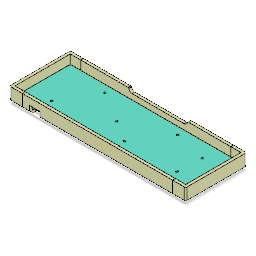
MiniVan_SpaceCut (Autodesk Fusion 360 design; units mm, degrees)
Autodesk Fusion 360 part; units mm, degrees
(part 1 of 4)
sketch "minivan_universal_plate_mount" plane through (80, 0, 0) normal (0, 1, 0) x (1, 0, 0)
  line L0 (-146.007, 0.6305) -> (-145.207, 0.6305)
  line L1 (-20.869, -43.7204) -> (-21.6683, -43.7204)
  line L2 (-243.231, -56.6448) -> (-243.231, 13.555101)
  line L3 (-146.007, 2.3007) -> (-146.007, 0.6305)
  line L4 (-137.022586, -19.0203) -> (-131.206, -19.0203)
  line L5 (-4.20028, -37.4695) -> (-4.20028, -24.6704)
  line L6 (-2.61827, -56.5195) -> (-1.81901, -56.5195)
  line L7 (-130.405, 0.6305) -> (-130.405, 2.3007)
  line L8 (-154.307, 7.53034) -> (-154.307, 4.7302)
  line L9 (-1.81901, -43.7204) -> (-2.61827, -43.7204)
  line L10 (-19.0004, -38.0703) -> (-4.99953, -38.0703)
  line L11 (-131.207, 0.6305) -> (-130.405, 0.6305)
  arc A0 (-243.231, 13.555101) -> (-240.231, 16.555101) centre (-240.231, 13.555101) cw
  line L12 (-153.432, 1.3) -> (-151.806, 1.3)
  line L13 (-130.405, -5.6203) -> (-131.206, -5.6203)
  line L14 (-17.4184, -56.5195) -> (-16.6192, -56.5195)
  line L15 (-151.806, 14.78019) -> (-151.806, 14.0004)
  line L16 (-1.81901, -56.5195) -> (-1.81901, -43.7204)
  line L17 (-145.205, -5.6203) -> (-146.006, -5.6203)
  line L18 (-151.806, 1.3) -> (-151.806, 0.1795)
  line L19 (-129.632, 1.3) -> (-127.905, 1.3)
  line L20 (-4.99953, -24.6704) -> (-4.99953, -24.0696)
  line L21 (-19.7997, -24.6704) -> (-19.7997, -37.4695)
  line L22 (-35.669, -43.7204) -> (-36.4684, -43.7204)
  line L23 (-24.5622, -18.4195) -> (-23.7629, -18.4195)
  line L24 (-9.76341, -19.0203) -> (-9.76341, -18.4195)
  line L25 (-19.0004, -37.4695) -> (-19.0004, -38.0703)
  line L26 (-36.4684, -43.7204) -> (-36.4684, -56.5195)
  line L27 (-36.4684, -56.5195) -> (-35.669, -56.5195)
  line L28 (-23.7629, -5.6203) -> (-24.5622, -5.6203)
  line L29 (-8.96278, -18.4195) -> (-8.96278, -5.6203)
  line L30 (-40.4301, -24.6704) -> (-41.2309, -24.6704)
  line L31 (-21.6683, -43.7204) -> (-21.6683, -43.1196)
  line L32 (-19.0004, -24.0696) -> (-19.0004, -24.6704)
  line L33 (-9.76341, -5.6203) -> (-9.76341, -5.0195)
  line L34 (-21.6683, -43.1196) -> (-30.570286, -43.1196)
  line L35 (-4.99953, -24.0696) -> (-19.0004, -24.0696)
  arc A1 (-30.570286, -42.918008) -> (-30.570286, -38.271592) centre (-31.493707, -40.5948) ccw
  line L36 (-25.6301, -24.6704) -> (-26.4308, -24.6704)
  line L37 (-26.4308, -24.0696) -> (-40.4301, -24.0696)
  line L38 (-21.6683, -56.5195) -> (-20.869, -56.5195)
  line L39 (-32.417127, -42.918008) -> (-32.417127, -43.1196)
  line L40 (-9.76341, -18.4195) -> (-8.96278, -18.4195)
  line L41 (-4.20028, -24.6704) -> (-4.99953, -24.6704)
  line L42 (-19.7997, -37.4695) -> (-19.0004, -37.4695)
  line L43 (-30.570286, -38.271592) -> (-30.570286, -38.0703)
  line L44 (-23.7629, -19.0203) -> (-9.76341, -19.0203)
  line L45 (-8.96278, -5.6203) -> (-9.76341, -5.6203)
  line L46 (-30.570286, -43.1196) -> (-30.570286, -42.918008)
  line L47 (-35.669, -56.5195) -> (-35.669, -57.1203)
  line L48 (-32.417127, -43.1196) -> (-35.669, -43.1196)
  line L49 (-24.5622, -5.6203) -> (-24.5622, -18.4195)
  line L50 (-30.570286, -38.0703) -> (-26.4308, -38.0703)
  line L51 (-26.4308, -37.4695) -> (-25.6301, -37.4695)
  line L52 (-4.99953, -38.0703) -> (-4.99953, -37.4695)
  line L53 (-9.76341, -5.0195) -> (-23.7629, -5.0195)
  line L54 (-26.4308, -38.0703) -> (-26.4308, -37.4695)
  line L55 (-21.6683, -57.1203) -> (-21.6683, -56.5195)
  line L56 (-25.6301, -37.4695) -> (-25.6301, -24.6704)
  line L57 (-35.669, -43.1196) -> (-35.669, -43.7204)
  line L58 (-35.669, -57.1203) -> (-21.6683, -57.1203)
  line L59 (-40.4301, -24.0696) -> (-40.4301, -24.6704)
  line L60 (-23.7629, -5.0195) -> (-23.7629, -5.6203)
  line L61 (-23.7629, -18.4195) -> (-23.7629, -19.0203)
  line L62 (-26.4308, -24.6704) -> (-26.4308, -24.0696)
  line L63 (-20.869, -56.5195) -> (-20.869, -43.7204)
  line L64 (-4.99953, -37.4695) -> (-4.20028, -37.4695)
  line L65 (-74.5684, -56.5195) -> (-73.769, -56.5195)
  line L66 (-82.7814, -37.4695) -> (-82.7814, -24.6704)
  arc A2 (-32.417127, -38.271592) -> (-32.417127, -42.918008) centre (-31.493707, -40.5948) ccw
  line L67 (-55.397707, 0.6305) -> (-54.598707, 0.6305)
  line L68 (-45.4822, -38.0703) -> (-45.4822, -37.4695)
  line L69 (-55.0058, -19.0203) -> (-55.0058, -18.4195)
  line L70 (-54.719, -56.5195) -> (-54.719, -57.1203)
  line L71 (-54.598707, 0.6305) -> (-54.598707, 0)
  line L72 (-35.1551, -18.4195) -> (-35.1551, -5.6203)
  line L73 (-49.9551, -19.0203) -> (-35.9558, -19.0203)
  line L74 (-54.719, -57.1203) -> (-40.7183, -57.1203)
  line L75 (-21.627707, 0.6305) -> (-20.828707, 0.6305)
  line L76 (-35.9558, -18.4195) -> (-35.1551, -18.4195)
  line L77 (-88.0551, -5.6203) -> (-88.8559, -5.6203)
  line L78 (-54.598707, 0) -> (-21.627707, 0)
  line L79 (-20.828707, 0.6305) -> (-20.828707, 13.42971)
  line L80 (-55.397707, 13.42971) -> (-55.397707, 0.6305)
  line L81 (-83.5808, -24.6704) -> (-83.5808, -24.0696)
  line L82 (-54.598707, 14.03054) -> (-54.598707, 13.42971)
  line L83 (-49.9551, -18.4195) -> (-49.9551, -19.0203)
  line L84 (-35.1551, -5.6203) -> (-35.9558, -5.6203)
  line L85 (-21.627707, 13.42971) -> (-21.627707, 14.03054)
  line L86 (-32.417127, -38.0703) -> (-32.417127, -38.271592)
  line L87 (-73.769, -56.5195) -> (-73.769, -57.1203)
  line L88 (-55.5184, -56.5195) -> (-54.719, -56.5195)
  line L89 (-55.0058, -18.4195) -> (-54.205, -18.4195)
  line L90 (-40.7183, -43.7204) -> (-40.7183, -43.1196)
  line L91 (-60.2823, -37.4695) -> (-59.4815, -37.4695)
  line L92 (-97.5801, -37.4695) -> (-97.5801, -38.0703)
  line L93 (-50.7559, -18.4195) -> (-49.9551, -18.4195)
  line L94 (-45.4822, -37.4695) -> (-44.6814, -37.4695)
  line L95 (-41.2309, -24.6704) -> (-41.2309, -37.4695)
  line L96 (-55.5184, -43.7204) -> (-55.5184, -56.5195)
  line L97 (-44.6814, -37.4695) -> (-44.6814, -24.6704)
  line L98 (-35.9558, -5.6203) -> (-35.9558, -5.0195)
  line L99 (-44.6814, -24.6704) -> (-45.4822, -24.6704)
  line L100 (-83.5808, -38.0703) -> (-83.5808, -37.4695)
  line L101 (-64.5322, -38.0703) -> (-64.5322, -37.4695)
  line L102 (-40.7183, -43.1196) -> (-54.719, -43.1196)
  line L103 (-73.255, -18.4195) -> (-73.255, -5.6203)
  line L104 (-49.9551, -5.0195) -> (-49.9551, -5.6203)
  line L105 (-40.4301, -37.4695) -> (-40.4301, -38.0703)
  line L106 (-49.9551, -5.6203) -> (-50.7559, -5.6203)
  line L107 (-39.9189, -43.7204) -> (-40.7183, -43.7204)
  line L108 (-21.627707, 0) -> (-21.627707, 0.6305)
  line L109 (-40.7183, -56.5195) -> (-39.9189, -56.5195)
  line L110 (-54.598707, 13.42971) -> (-55.397707, 13.42971)
  line L111 (-21.627707, 14.03054) -> (-54.598707, 14.03054)
  line L112 (-92.819, -57.1203) -> (-78.8183, -57.1203)
  line L113 (-50.7559, -5.6203) -> (-50.7559, -18.4195)
  line L114 (-41.2309, -37.4695) -> (-40.4301, -37.4695)
  line L115 (-35.9558, -19.0203) -> (-35.9558, -18.4195)
  line L116 (-54.719, -43.7204) -> (-55.5184, -43.7204)
  line L117 (-54.719, -43.1196) -> (-54.719, -43.7204)
  line L118 (-83.5808, -37.4695) -> (-82.7814, -37.4695)
  line L119 (-60.2823, -24.6704) -> (-60.2823, -37.4695)
  line L120 (-55.0058, -5.6203) -> (-55.0058, -5.0195)
  line L121 (-69.8059, -5.6203) -> (-69.8059, -18.4195)
  line L122 (-39.9189, -56.5195) -> (-39.9189, -43.7204)
  line L123 (-97.5801, -38.0703) -> (-83.5808, -38.0703)
  line L124 (-82.7814, -24.6704) -> (-83.5808, -24.6704)
  line L125 (-54.205, -5.6203) -> (-55.0058, -5.6203)
  line L126 (-54.205, -18.4195) -> (-54.205, -5.6203)
  line L127 (-98.3809, -37.4695) -> (-97.5801, -37.4695)
  line L128 (-97.5801, -24.0696) -> (-97.5801, -24.6704)
  line L129 (-59.7683, -57.1203) -> (-59.7683, -56.5195)
  line L130 (-69.0051, -5.0195) -> (-69.0051, -5.6203)
  line L131 (-73.255, -5.6203) -> (-74.0558, -5.6203)
  line L132 (-58.9689, -43.7204) -> (-59.7683, -43.7204)
  line L133 (-74.0558, -5.6203) -> (-74.0558, -5.0195)
  line L134 (-73.769, -43.1196) -> (-73.769, -43.7204)
  line L135 (-74.0558, -18.4195) -> (-73.255, -18.4195)
  line L136 (-78.5315, -24.6704) -> (-79.3309, -24.6704)
  line L137 (-92.819, -43.7204) -> (-93.6184, -43.7204)
  line L138 (-79.3309, -24.6704) -> (-79.3309, -37.4695)
  line L139 (-78.0189, -43.7204) -> (-78.8183, -43.7204)
  line L140 (-59.7683, -43.7204) -> (-59.7683, -43.1196)
  line L141 (-107.906, -5.6203) -> (-107.906, -18.4195)
  line L142 (-79.3309, -37.4695) -> (-78.5315, -37.4695)
  line L143 (-88.0551, -19.0203) -> (-74.0558, -19.0203)
  line L144 (-64.5322, -37.4695) -> (-63.7314, -37.4695)
  line L145 (-83.5808, -24.0696) -> (-97.5801, -24.0696)
  line L146 (-107.105, -5.6203) -> (-107.906, -5.6203)
  line L147 (-58.9689, -56.5195) -> (-58.9689, -43.7204)
  line L148 (-73.769, -57.1203) -> (-59.7683, -57.1203)
  line L149 (-93.6184, -43.7204) -> (-93.6184, -56.5195)
  line L150 (-64.5322, -24.0696) -> (-78.5315, -24.0696)
  line L151 (-74.0558, -5.0195) -> (-88.0551, -5.0195)
  line L152 (-78.8183, -43.7204) -> (-78.8183, -43.1196)
  line L153 (-63.7314, -37.4695) -> (-63.7314, -24.6704)
  line L154 (-74.5684, -43.7204) -> (-74.5684, -56.5195)
  line L155 (-78.5315, -37.4695) -> (-78.5315, -38.0703)
  line L156 (-64.5322, -24.6704) -> (-64.5322, -24.0696)
  line L157 (-88.0551, -5.0195) -> (-88.0551, -5.6203)
  line L158 (-88.0551, -18.4195) -> (-88.0551, -19.0203)
  line L159 (-88.8559, -18.4195) -> (-88.0551, -18.4195)
  line L160 (-108.825381, -38.0703) -> (-108.825381, -38.365605)
  line L161 (-116.918, -43.7204) -> (-116.918, -43.1196)
  line L162 (-78.8183, -57.1203) -> (-78.8183, -56.5195)
  line L163 (-116.918, -57.1203) -> (-116.918, -56.5195)
  line L164 (-101.83, -37.4695) -> (-101.83, -24.6704)
  line L165 (-126.155, -5.0195) -> (-126.155, -5.6203)
  line L166 (-116.119, -56.5195) -> (-116.119, -43.7204)
  line L167 (-131.718, -56.5195) -> (-130.919, -56.5195)
  line L168 (-97.8683, -43.1196) -> (-106.562032, -43.1196)
  line L169 (-126.956, -5.6203) -> (-126.956, -18.4195)
  line L170 (-93.1058, -18.4195) -> (-92.305, -18.4195)
  line L171 (-112.156, -19.0203) -> (-112.156, -18.4195)
  line L172 (-108.825381, -43.1196) -> (-111.869, -43.1196)
  line L173 (-92.819, -56.5195) -> (-92.819, -57.1203)
  line L174 (-117.431, -37.4695) -> (-116.63, -37.4695)
  line L175 (-74.0558, -19.0203) -> (-74.0558, -18.4195)
  line L176 (-130.919, -57.1203) -> (-116.918, -57.1203)
  line L177 (-92.819, -43.1196) -> (-92.819, -43.7204)
  line L178 (-107.906, -18.4195) -> (-107.105, -18.4195)
  line L179 (-98.3809, -24.6704) -> (-98.3809, -37.4695)
  line L180 (-111.869, -43.1196) -> (-111.869, -43.7204)
  line L181 (-111.869, -57.1203) -> (-97.8683, -57.1203)
  line L182 (-130.919, -43.7204) -> (-131.718, -43.7204)
  line L183 (-78.5315, -38.0703) -> (-64.5322, -38.0703)
  line L184 (-112.156, -5.0195) -> (-126.155, -5.0195)
  line L185 (-63.7314, -24.6704) -> (-64.5322, -24.6704)
  line L186 (-55.0058, -5.0195) -> (-69.0051, -5.0195)
  line L187 (-112.156, -18.4195) -> (-111.355, -18.4195)
  line L188 (-130.919, -56.5195) -> (-130.919, -57.1203)
  line L189 (-78.0189, -56.5195) -> (-78.0189, -43.7204)
  line L190 (-111.355, -18.4195) -> (-111.355, -5.6203)
  line L191 (-111.355, -5.6203) -> (-112.156, -5.6203)
  line L192 (-116.918, -56.5195) -> (-116.119, -56.5195)
  line L193 (-97.0689, -43.7204) -> (-97.8683, -43.7204)
  line L194 (-117.431, -24.6704) -> (-117.431, -37.4695)
  line L195 (-107.105, -19.0203) -> (-93.1058, -19.0203)
  line L196 (-97.5801, -24.6704) -> (-98.3809, -24.6704)
  line L197 (-106.562032, -43.1196) -> (-106.562032, -42.823995)
  line L198 (-78.8183, -56.5195) -> (-78.0189, -56.5195)
  line L199 (-73.769, -43.7204) -> (-74.5684, -43.7204)
  line L200 (-88.8559, -5.6203) -> (-88.8559, -18.4195)
  line L201 (-131.718, -43.7204) -> (-131.718, -56.5195)
  line L202 (-78.5315, -24.0696) -> (-78.5315, -24.6704)
  line L203 (-93.6184, -56.5195) -> (-92.819, -56.5195)
  line L204 (-93.1058, -5.0195) -> (-107.105, -5.0195)
  line L205 (-59.7683, -43.1196) -> (-73.769, -43.1196)
  line L206 (-116.63, -37.4695) -> (-116.63, -38.0703)
  line L207 (-112.668, -43.7204) -> (-112.668, -56.5195)
  arc A3 (-108.825381, -38.365605) -> (-108.825381, -42.823995) centre (-107.693707, -40.5948) ccw
  line L208 (-107.105, -18.4195) -> (-107.105, -19.0203)
  line L209 (-59.7683, -56.5195) -> (-58.9689, -56.5195)
  line L210 (-106.562032, -38.0703) -> (-102.631, -38.0703)
  line L211 (-102.631, -37.4695) -> (-101.83, -37.4695)
  line L212 (-116.63, -24.6704) -> (-117.431, -24.6704)
  line L213 (-106.562032, -38.365605) -> (-106.562032, -38.0703)
  line L214 (-108.825381, -42.823995) -> (-108.825381, -43.1196)
  line L215 (-78.8183, -43.1196) -> (-92.819, -43.1196)
  line L216 (-112.156, -5.6203) -> (-112.156, -5.0195)
  line L217 (-107.105, -5.0195) -> (-107.105, -5.6203)
  line L218 (-111.869, -43.7204) -> (-112.668, -43.7204)
  line L219 (-111.869, -56.5195) -> (-111.869, -57.1203)
  line L220 (-97.8683, -56.5195) -> (-97.0689, -56.5195)
  line L221 (-116.119, -43.7204) -> (-116.918, -43.7204)
  line L222 (-97.8683, -57.1203) -> (-97.8683, -56.5195)
  line L223 (-121.682, -37.4695) -> (-120.881, -37.4695)
  line L224 (-150.768, -56.5195) -> (-149.969, -56.5195)
  line L225 (-164.255, -5.0195) -> (-164.255, -5.6203)
  line L226 (-121.682, -38.0703) -> (-121.682, -37.4695)
  line L227 (-155.018, -43.1196) -> (-169.019, -43.1196)
  line L228 (-135.169, -56.5195) -> (-135.169, -43.7204)
  line L229 (-102.631, -24.0696) -> (-116.63, -24.0696)
  line L230 (-169.818, -56.5195) -> (-169.019, -56.5195)
  line L231 (-116.918, -43.1196) -> (-130.919, -43.1196)
  line L232 (-154.732, -37.4695) -> (-154.732, -38.0703)
  line L233 (-154.732, -24.6704) -> (-155.532, -24.6704)
  line L234 (-116.63, -38.0703) -> (-108.825381, -38.0703)
  line L235 (-101.83, -24.6704) -> (-102.631, -24.6704)
  line L236 (-135.682, -24.6704) -> (-136.482, -24.6704)
  line L237 (-97.8683, -43.7204) -> (-97.8683, -43.1196)
  line L238 (-164.255, -19.0203) -> (-150.256, -19.0203)
  line L239 (-126.155, -18.4195) -> (-126.155, -19.0203)
  line L240 (-97.0689, -56.5195) -> (-97.0689, -43.7204)
  line L241 (-116.63, -24.0696) -> (-116.63, -24.6704)
  line L242 (-150.256, -5.6203) -> (-150.256, -5.0195)
  line L243 (-169.818, -43.7204) -> (-169.818, -56.5195)
  line L244 (-135.682, -24.0696) -> (-135.682, -24.6704)
  line L245 (-154.219, -43.7204) -> (-155.018, -43.7204)
  line L246 (-139.931, -37.4695) -> (-139.931, -24.6704)
  line L247 (-135.968, -57.1203) -> (-135.968, -56.5195)
  line L248 (-169.019, -43.1196) -> (-169.019, -43.7204)
  line L249 (-150.256, -18.4195) -> (-149.455, -18.4195)
  line L250 (-112.668, -56.5195) -> (-111.869, -56.5195)
  line L251 (-93.1058, -5.6203) -> (-93.1058, -5.0195)
  line L252 (-92.305, -5.6203) -> (-93.1058, -5.6203)
  line L253 (-169.019, -43.7204) -> (-169.818, -43.7204)
  line L254 (-102.631, -24.6704) -> (-102.631, -24.0696)
  line L255 (-93.1058, -19.0203) -> (-93.1058, -18.4195)
  line L256 (-149.969, -57.1203) -> (-135.968, -57.1203)
  line L257 (-126.155, -5.6203) -> (-126.956, -5.6203)
  line L258 (-149.969, -43.1196) -> (-149.969, -43.7204)
  line L259 (-149.969, -56.5195) -> (-149.969, -57.1203)
  line L260 (-154.219, -56.5195) -> (-154.219, -43.7204)
  line L261 (-135.968, -43.1196) -> (-149.969, -43.1196)
  line L262 (-155.018, -43.7204) -> (-155.018, -43.1196)
  line L263 (-155.018, -56.5195) -> (-154.219, -56.5195)
  line L264 (-121.682, -24.0696) -> (-135.682, -24.0696)
  line L265 (-140.732, -24.6704) -> (-140.732, -24.0696)
  line L266 (-135.968, -56.5195) -> (-135.169, -56.5195)
  line L267 (-120.881, -24.6704) -> (-121.682, -24.6704)
  line L268 (-173.782, -24.6704) -> (-174.582, -24.6704)
  line L269 (-135.169, -43.7204) -> (-135.968, -43.7204)
  line L270 (-92.305, -18.4195) -> (-92.305, -5.6203)
  line L271 (-126.956, -18.4195) -> (-126.155, -18.4195)
  line L272 (-102.631, -38.0703) -> (-102.631, -37.4695)
  line L273 (-149.455, -18.4195) -> (-149.455, -5.6203)
  line L274 (-155.018, -57.1203) -> (-155.018, -56.5195)
  line L275 (-150.768, -43.7204) -> (-150.768, -56.5195)
  line L276 (-126.155, -19.0203) -> (-112.156, -19.0203)
  line L277 (-169.019, -57.1203) -> (-155.018, -57.1203)
  line L278 (-174.582, -24.6704) -> (-174.582, -37.4695)
  arc A4 (-106.562032, -42.823995) -> (-106.562032, -38.365605) centre (-107.693707, -40.5948) ccw
  line L279 (-140.732, -38.0703) -> (-140.732, -37.4695)
  line L280 (-120.881, -37.4695) -> (-120.881, -24.6704)
  line L281 (-154.732, -38.0703) -> (-140.732, -38.0703)
  line L282 (-165.057, -18.4195) -> (-164.255, -18.4195)
  line L283 (-149.455, -5.6203) -> (-150.256, -5.6203)
  line L284 (-174.582, -37.4695) -> (-173.782, -37.4695)
  line L285 (-159.782, -24.0696) -> (-173.782, -24.0696)
  line L286 (-155.532, -37.4695) -> (-154.732, -37.4695)
  line L287 (-188.069, -56.5195) -> (-188.069, -57.1203)
  line L288 (-173.782, -38.0703) -> (-159.782, -38.0703)
  line L289 (-164.255, -18.4195) -> (-164.255, -19.0203)
  line L290 (-188.069, -43.1196) -> (-188.069, -43.7204)
  line L291 (-193.632, -24.6704) -> (-193.632, -37.4695)
  line L292 (-183.307, -19.0203) -> (-169.307, -19.0203)
  line L293 (-136.482, -37.4695) -> (-135.682, -37.4695)
  line L294 (-173.782, -37.4695) -> (-173.782, -38.0703)
  line L295 (-202.357, -5.6203) -> (-203.157, -5.6203)
  line L296 (-183.307, -18.4195) -> (-183.307, -19.0203)
  line L297 (-158.981, -37.4695) -> (-158.981, -24.6704)
  line L298 (-188.357, -5.0195) -> (-202.357, -5.0195)
  line L299 (-169.019, -56.5195) -> (-169.019, -57.1203)
  line L300 (-188.069, -57.1203) -> (-174.068, -57.1203)
  line L301 (-174.068, -43.1196) -> (-188.069, -43.1196)
  line L302 (-192.832, -24.0696) -> (-192.832, -24.6704)
  line L303 (-130.919, -43.1196) -> (-130.919, -43.7204)
  line L304 (-188.357, -19.0203) -> (-188.357, -18.4195)
  line L305 (-174.068, -56.5195) -> (-173.269, -56.5195)
  line L306 (-188.868, -43.7204) -> (-188.868, -56.5195)
  line L307 (-135.682, -38.0703) -> (-121.682, -38.0703)
  line L308 (-174.068, -43.7204) -> (-174.068, -43.1196)
  line L309 (-149.969, -43.7204) -> (-150.768, -43.7204)
  line L310 (-183.307, -5.6203) -> (-184.107, -5.6203)
  line L311 (-121.682, -24.6704) -> (-121.682, -24.0696)
  line L312 (-135.968, -43.7204) -> (-135.968, -43.1196)
  line L313 (-150.256, -19.0203) -> (-150.256, -18.4195)
  line L314 (-169.307, -5.6203) -> (-169.307, -5.0195)
  line L315 (-140.732, -24.0696) -> (-154.732, -24.0696)
  line L316 (-136.482, -24.6704) -> (-136.482, -37.4695)
  line L317 (-139.931, -24.6704) -> (-140.732, -24.6704)
  line L318 (-202.357, 0.0297) -> (-188.357, 0.0297)
  line L319 (-169.307, -18.4195) -> (-168.505, -18.4195)
  line L320 (-178.832, -24.6704) -> (-178.832, -24.0696)
  line L321 (-173.269, -43.7204) -> (-174.068, -43.7204)
  line L322 (-135.682, -37.4695) -> (-135.682, -38.0703)
  line L323 (-150.256, -5.0195) -> (-164.255, -5.0195)
  line L324 (-193.632, -37.4695) -> (-192.832, -37.4695)
  line L325 (-158.981, -24.6704) -> (-159.782, -24.6704)
  line L326 (-165.057, -5.6203) -> (-165.057, -18.4195)
  line L327 (-159.782, -38.0703) -> (-159.782, -37.4695)
  line L328 (-188.357, 0.0297) -> (-188.357, 0.6305)
  line L329 (-178.832, -38.0703) -> (-178.832, -37.4695)
  line L330 (-169.307, -5.0195) -> (-183.307, -5.0195)
  line L331 (-164.255, -5.6203) -> (-165.057, -5.6203)
  line L332 (-178.031, -37.4695) -> (-178.031, -24.6704)
  line L333 (-203.157, 13.42971) -> (-203.157, 0.6305)
  line L334 (-202.357, 13.42971) -> (-203.157, 13.42971)
  line L335 (-154.732, -24.0696) -> (-154.732, -24.6704)
  line L336 (-187.556, -18.4195) -> (-187.556, -5.6203)
  line L337 (-140.732, -37.4695) -> (-139.931, -37.4695)
  line L338 (-178.832, -24.0696) -> (-192.832, -24.0696)
  line L339 (-173.782, -24.0696) -> (-173.782, -24.6704)
  line L340 (-155.532, -24.6704) -> (-155.532, -37.4695)
  line L341 (-202.357, -5.0195) -> (-202.357, -5.6203)
  line L342 (-159.782, -24.6704) -> (-159.782, -24.0696)
  line L343 (-234.112, -56.5195) -> (-233.313, -56.5195)
  line L344 (-221.407, -5.6203) -> (-222.207, -5.6203)
  line L345 (-220.894, -37.4695) -> (-220.894, -24.6704)
  line L346 (-233.313, -43.7204) -> (-234.112, -43.7204)
  line L347 (-211.882, -24.6704) -> (-212.682, -24.6704)
  line L348 (-203.157, -18.4195) -> (-202.357, -18.4195)
  line L349 (-219.313, -43.7204) -> (-219.313, -43.1196)
  line L350 (-233.313, -43.1196) -> (-233.313, -43.7204)
  line L351 (-235.694, -37.4695) -> (-235.694, -38.0703)
  line L352 (-202.357, 14.03054) -> (-202.357, 13.42971)
  line L353 (-197.882, -24.6704) -> (-197.882, -24.0696)
  line L354 (-207.119, -57.1203) -> (-193.118, -57.1203)
  line L355 (-197.081, -37.4695) -> (-197.081, -24.6704)
  line L356 (-197.882, -38.0703) -> (-197.882, -37.4695)
  line L357 (-207.407, -19.0203) -> (-207.407, -18.4195)
  line L358 (-202.357, 0.6305) -> (-202.357, 0.0297)
  line L359 (-221.693, -37.4695) -> (-220.894, -37.4695)
  line L360 (-188.069, -43.7204) -> (-188.868, -43.7204)
  line L361 (-192.832, -38.0703) -> (-178.832, -38.0703)
  line L362 (-173.269, -56.5195) -> (-173.269, -43.7204)
  line L363 (-211.882, -24.0696) -> (-211.882, -24.6704)
  line L364 (-193.118, -57.1203) -> (-193.118, -56.5195)
  line L365 (-211.882, -37.4695) -> (-211.882, -38.0703)
  line L366 (-188.357, -18.4195) -> (-187.556, -18.4195)
  line L367 (-169.307, -19.0203) -> (-169.307, -18.4195)
  line L368 (-202.357, -18.4195) -> (-202.357, -19.0203)
  line L369 (-178.031, -24.6704) -> (-178.832, -24.6704)
  line L370 (-207.119, -56.5195) -> (-207.119, -57.1203)
  line L371 (-207.119, -43.1196) -> (-207.119, -43.7204)
  line L372 (-168.505, -5.6203) -> (-169.307, -5.6203)
  line L373 (-192.832, -24.6704) -> (-193.632, -24.6704)
  line L374 (-174.068, -57.1203) -> (-174.068, -56.5195)
  line L375 (-184.107, -5.6203) -> (-184.107, -18.4195)
  line L376 (-193.118, -56.5195) -> (-192.319, -56.5195)
  line L377 (-188.357, 14.03054) -> (-202.357, 14.03054)
  line L378 (-235.694, -38.0703) -> (-221.693, -38.0703)
  line L379 (-192.832, -37.4695) -> (-192.832, -38.0703)
  line L380 (-193.118, -43.7204) -> (-193.118, -43.1196)
  line L381 (-206.606, -5.6203) -> (-207.407, -5.6203)
  line L382 (-202.357, -19.0203) -> (-188.357, -19.0203)
  line L383 (-203.157, 0.6305) -> (-202.357, 0.6305)
  line L384 (-197.882, -24.0696) -> (-211.882, -24.0696)
  line L385 (-178.832, -37.4695) -> (-178.031, -37.4695)
  line L386 (-203.157, -5.6203) -> (-203.157, -18.4195)
  line L387 (-221.407, -19.0203) -> (-207.407, -19.0203)
  line L388 (-187.556, -5.6203) -> (-188.357, -5.6203)
  line L389 (-221.407, -5.0195) -> (-221.407, -5.6203)
  line L390 (-221.693, -38.0703) -> (-221.693, -37.4695)
  line L391 (-207.407, -5.0195) -> (-221.407, -5.0195)
  line L392 (-187.556, 13.42971) -> (-188.357, 13.42971)
  line L393 (-188.357, -5.6203) -> (-188.357, -5.0195)
  line L394 (-159.782, -37.4695) -> (-158.981, -37.4695)
  line L395 (-219.313, -56.5195) -> (-218.513, -56.5195)
  line L396 (-236.493, -24.6704) -> (-236.493, -37.4695)
  line L397 (-207.119, -43.7204) -> (-207.918, -43.7204)
  line L398 (-218.513, -43.7204) -> (-219.313, -43.7204)
  line L399 (-183.307, -5.0195) -> (-183.307, -5.6203)
  line L400 (-188.868, -56.5195) -> (-188.069, -56.5195)
  line L401 (-212.682, -24.6704) -> (-212.682, -37.4695)
  line L402 (-235.694, -24.6704) -> (-236.493, -24.6704)
  line L403 (-212.682, -37.4695) -> (-211.882, -37.4695)
  line L404 (-168.505, -18.4195) -> (-168.505, -5.6203)
  line L405 (-184.107, -18.4195) -> (-183.307, -18.4195)
  line L406 (-234.112, -43.7204) -> (-234.112, -56.5195)
  line L407 (-235.694, -24.0696) -> (-235.694, -24.6704)
  line L408 (-206.606, 0.6305) -> (-206.606, 13.42971)
  line L409 (-226.457, 14) -> (-226.457, 14.03054)
  line L410 (-187.556, 0.6305) -> (-187.556, 13.42971)
  line L411 (-188.357, 13.42971) -> (-188.357, 14.03054)
  line L412 (-226.457, -5.0195) -> (-240.457, -5.0195)
  line L413 (-57.3885, 14.03054) -> (-73.608707, 14.03054)
  line L414 (-2.617707, 14) -> (-4.99953, 14)
  line L415 (-2.617707, 0.0297) -> (-2.617707, 0.6305)
  line L416 (-2.617707, 0.6305) -> (-1.818707, 0.6305)
  line L417 (-220.894, -24.6704) -> (-221.693, -24.6704)
  line L418 (-207.407, 13.42971) -> (-207.407, 14.03054)
  line L419 (-192.319, -43.7204) -> (-193.118, -43.7204)
  line L420 (-206.606, -18.4195) -> (-206.606, -5.6203)
  line L421 (-188.357, 0.6305) -> (-187.556, 0.6305)
  line L422 (-219.313, -43.1196) -> (-233.313, -43.1196)
  line L423 (-197.882, -37.4695) -> (-197.081, -37.4695)
  line L424 (-193.118, -43.1196) -> (-207.119, -43.1196)
  line L425 (-222.207, -5.6203) -> (-222.207, -18.4195)
  line L426 (-240.457, 14.03054) -> (-240.457, 13.42971)
  line L427 (-206.606, 13.42971) -> (-207.407, 13.42971)
  line L428 (-211.882, -38.0703) -> (-197.882, -38.0703)
  line L429 (-226.457, -5.6203) -> (-226.457, -5.0195)
  line L430 (-225.656, -18.4195) -> (-225.656, -5.6203)
  line L431 (-207.407, 14.03054) -> (-221.407, 14.03054)
  line L432 (-197.081, -24.6704) -> (-197.882, -24.6704)
  line L433 (-226.457, -18.4195) -> (-225.656, -18.4195)
  line L434 (-240.457, -5.6203) -> (-241.257, -5.6203)
  line L435 (-218.513, -56.5195) -> (-218.513, -43.7204)
  line L436 (-240.457, 0.6305) -> (-240.457, 0.0297)
  line L437 (-219.313, -57.1203) -> (-219.313, -56.5195)
  line L438 (-240.457, -18.4195) -> (-240.457, -19.0203)
  line L439 (-192.319, -56.5195) -> (-192.319, -43.7204)
  line L440 (-221.407, -18.4195) -> (-221.407, -19.0203)
  line L441 (-221.407, 14) -> (-226.457, 14)
  line L442 (-226.457, -19.0203) -> (-226.457, -18.4195)
  line L443 (-236.493, -37.4695) -> (-235.694, -37.4695)
  line L444 (-207.918, -43.7204) -> (-207.918, -56.5195)
  line L445 (-233.313, -56.5195) -> (-233.313, -57.1203)
  line L446 (-233.313, -57.1203) -> (-219.313, -57.1203)
  line L447 (-241.257, 0.6305) -> (-240.457, 0.6305)
  line L448 (-221.693, -24.0696) -> (-235.694, -24.0696)
  line L449 (-241.257, -5.6203) -> (-241.257, -18.4195)
  line L450 (-221.407, 14.03054) -> (-221.407, 14)
  line L451 (-240.457, 13.42971) -> (-241.257, 13.42971)
  line L452 (-207.407, 0.0297) -> (-207.407, 0.6305)
  line L453 (-226.457, 14.03054) -> (-240.457, 14.03054)
  line L454 (-241.257, -18.4195) -> (-240.457, -18.4195)
  line L455 (-74.407707, 8.205101) -> (-76.843707, 8.205101)
  line L456 (-161.363, 0.6305) -> (-161.363, 13.42971)
  line L457 (-207.918, -56.5195) -> (-207.119, -56.5195)
  line L458 (-207.407, 0.6305) -> (-206.606, 0.6305)
  line L459 (-221.693, -24.6704) -> (-221.693, -24.0696)
  line L460 (-207.407, -18.4195) -> (-206.606, -18.4195)
  circle A5 centre (-182.431, 5.905101) radius 2.5
  line L461 (-222.207, -18.4195) -> (-221.407, -18.4195)
  line L462 (-240.457, 0.0297) -> (-207.407, 0.0297)
  line L463 (-207.407, -5.6203) -> (-207.407, -5.0195)
  line L464 (-240.457, -19.0203) -> (-226.457, -19.0203)
  line L465 (-225.656, -5.6203) -> (-226.457, -5.6203)
  line L466 (-240.457, -5.0195) -> (-240.457, -5.6203)
  line L467 (-241.257, 13.42971) -> (-241.257, 0.6305)
  circle A6 centre (-29.943707, -5.844899) radius 2.5
  circle A7 centre (-210.731, -42.8948) radius 2.5
  line L468 (-56.5877, 0.6305) -> (-56.5877, 13.42971)
  line L469 (-164.543, 14) -> (-164.543, 14.03054)
  line L470 (-162.162, 14) -> (-164.543, 14)
  line L471 (-19.0004, 0.6305) -> (-19.0004, 0.0297)
  line L472 (-73.608707, 13.42971) -> (-74.407707, 13.42971)
  line L473 (-4.99953, 14) -> (-4.99953, 14.03054)
  line L474 (-105.525, 0.6305) -> (-104.725, 0.6305)
  line L475 (-19.7997, 13.42971) -> (-19.7997, 0.6305)
  line L476 (-57.3885, 13.42971) -> (-57.3885, 14.03054)
  line L477 (-82.5003, 1.3) -> (-82.5003, 4.7302)
  line L478 (-19.7997, 0.6305) -> (-19.0004, 0.6305)
  line L479 (-1.818707, 13.42971) -> (-2.617707, 13.42971)
  line L480 (-162.162, 13.42971) -> (-162.162, 14)
  line L481 (-105.525, 2.3007) -> (-105.525, 0.6305)
  line L482 (-131.207, 13.42971) -> (-131.207, 14.03054)
  line L483 (-108.024, 1.3) -> (-106.299, 1.3)
  line L484 (-111.325, 0.1795) -> (-108.024, 0.1795)
  line L485 (-89.1494, 2.3007) -> (-89.1494, 1.3)
  line L486 (-106.299, 2.3007) -> (-105.525, 2.3007)
  line L487 (-74.407707, 13.42971) -> (-74.407707, 8.205101)
  line L488 (-108.024, 0.1795) -> (-108.024, 1.3)
  line L489 (-90.7246, 0.6305) -> (-89.9252, 0.6305)
  line L490 (-178.544, 0.0297) -> (-162.162, 0.0297)
  line L491 (-1.818707, 0.6305) -> (-1.818707, 13.42971)
  line L492 (-76.843707, 3.205101) -> (-74.407707, 3.205101)
  line L493 (-90.7246, 0.0297) -> (-90.7246, 0.6305)
  line L494 (-178.544, 14.03054) -> (-178.544, 13.42971)
  line L495 (-56.5877, 13.42971) -> (-57.3885, 13.42971)
  line L496 (-162.162, 0.0297) -> (-162.162, 0.6305)
  line L497 (-179.343, 13.42971) -> (-179.343, 0.6305)
  line L498 (-87.424, 14.78019) -> (-87.424, 14.0004)
  line L499 (-90.7246, 13.42971) -> (-90.7246, 14.03054)
  line L500 (-4.99953, 14.03054) -> (-19.0004, 14.03054)
  arc A8 (-76.843707, 8.205101) -> (-76.843707, 3.205101) centre (-76.843707, 5.705101) ccw
  line L501 (-19.0004, 0.0297) -> (-2.617707, 0.0297)
  line L502 (-57.3885, 0.0297) -> (-57.3885, 0.6305)
  line L503 (-129.632, 12.99978) -> (-130.405, 12.99978)
  line L504 (-130.405, 12.99978) -> (-130.405, 13.42971)
  line L505 (-104.725, 0.6305) -> (-104.725, 0.0297)
  line L506 (-124.606, 14.78019) -> (-127.905, 14.78019)
  line L507 (-111.325, 1.3) -> (-111.325, 0.1795)
  line L508 (-178.544, 0.6305) -> (-178.544, 0.0297)
  line L509 (-106.299, 1.3) -> (-106.299, 2.3007)
  line L510 (-89.9252, 0.6305) -> (-89.9252, 2.3007)
  line L511 (-178.544, 13.42971) -> (-179.343, 13.42971)
  line L512 (-2.617707, 13.42971) -> (-2.617707, 14)
  line L513 (-19.0004, 14.03054) -> (-19.0004, 13.42971)
  line L514 (-73.608707, 0.6305) -> (-73.608707, 0.0297)
  line L515 (-161.363, 13.42971) -> (-162.162, 13.42971)
  line L516 (-164.543, 14.03054) -> (-178.544, 14.03054)
  line L517 (-179.343, 0.6305) -> (-178.544, 0.6305)
  line L518 (-74.407707, 0.6305) -> (-73.608707, 0.6305)
  line L519 (-19.0004, 13.42971) -> (-19.7997, 13.42971)
  line L520 (-73.608707, 14.03054) -> (-73.608707, 13.42971)
  line L521 (-162.162, 0.6305) -> (-161.363, 0.6305)
  line L522 (-111.325, 14.0004) -> (-112.95, 14.0004)
  line L523 (-57.3885, 0.6305) -> (-56.5877, 0.6305)
  line L524 (-74.407707, 3.205101) -> (-74.407707, 0.6305)
  line L525 (-73.608707, 0.0297) -> (-57.3885, 0.0297)
  line L526 (-127.905, 14.0004) -> (-129.632, 14.0004)
  line L527 (-84.1252, 14.0004) -> (-84.1252, 14.78019)
  line L528 (-90.7246, 14.03054) -> (-104.725, 14.03054)
  line L529 (-104.725, 0.0297) -> (-90.7246, 0.0297)
  line L530 (-131.207, 14.03054) -> (-145.207, 14.03054)
  line L531 (-108.024, 14.0004) -> (-108.024, 14.78019)
  line L532 (-89.9252, 2.3007) -> (-89.1494, 2.3007)
  line L533 (-111.325, 14.78019) -> (-111.325, 14.0004)
  line L534 (-122.107, 4.7302) -> (-122.107, 7.53034)
  line L535 (-112.95, 4.7302) -> (-112.95, 1.3)
  line L536 (-127.905, 14.78019) -> (-127.905, 14.0004)
  line L537 (-122.982, 7.53034) -> (-122.982, 14.0004)
  line L538 (-124.606, 0.1795) -> (-124.606, 1.3)
  line L539 (-105.525, 12.99978) -> (-106.299, 12.99978)
  line L540 (-89.9252, 13.42971) -> (-90.7246, 13.42971)
  line L541 (-145.207, 13.42971) -> (-146.007, 13.42971)
  line L542 (-81.6254, 7.53034) -> (-82.5003, 7.53034)
  line L543 (-84.1252, 0.1795) -> (-84.1252, 1.3)
  line L544 (-112.95, 7.53034) -> (-113.824, 7.53034)
  line L545 (-112.95, 14.0004) -> (-112.95, 7.53034)
  line L546 (-82.5003, 4.7302) -> (-81.6254, 4.7302)
  line L547 (-108.024, 14.78019) -> (-111.325, 14.78019)
  line L548 (-146.007, 12.99978) -> (-146.782, 12.99978)
  line L549 (-104.725, 14.03054) -> (-104.725, 13.42971)
  line L550 (-106.299, 14.0004) -> (-108.024, 14.0004)
  line L551 (-84.1252, 1.3) -> (-82.5003, 1.3)
  line L552 (-127.905, 0.1795) -> (-124.606, 0.1795)
  line L553 (-124.606, 1.3) -> (-122.982, 1.3)
  line L554 (-89.9252, 12.99978) -> (-89.9252, 13.42971)
  line L555 (-127.905, 1.3) -> (-127.905, 0.1795)
  line L556 (-145.207, 14.03054) -> (-145.207, 13.42971)
  line L557 (-146.782, 12.99978) -> (-146.782, 14.0004)
  line L558 (-82.5003, 7.53034) -> (-82.5003, 14.0004)
  line L559 (-82.5003, 14.0004) -> (-84.1252, 14.0004)
  line L560 (-89.1494, 1.3) -> (-87.424, 1.3)
  line L561 (-113.824, 4.7302) -> (-112.95, 4.7302)
  line L562 (-146.007, 13.42971) -> (-146.007, 12.99978)
  line L563 (-130.405, 13.42971) -> (-131.207, 13.42971)
  line L564 (-113.824, 7.53034) -> (-113.824, 4.7302)
  line L565 (-87.424, 0.1795) -> (-84.1252, 0.1795)
  line L566 (-84.1252, 14.78019) -> (-87.424, 14.78019)
  line L567 (-87.424, 1.3) -> (-87.424, 0.1795)
  line L568 (-87.424, 14.0004) -> (-89.1494, 14.0004)
  line L569 (-112.95, 1.3) -> (-111.325, 1.3)
  line L570 (-81.6254, 4.7302) -> (-81.6254, 7.53034)
  line L571 (-106.299, 12.99978) -> (-106.299, 14.0004)
  line L572 (-122.982, 1.3) -> (-122.982, 4.7302)
  line L573 (-124.606, 14.0004) -> (-124.606, 14.78019)
  line L574 (-89.1494, 12.99978) -> (-89.9252, 12.99978)
  line L575 (-105.525, 13.42971) -> (-105.525, 12.99978)
  line L576 (-122.982, 14.0004) -> (-124.606, 14.0004)
  line L577 (-145.205, -5.0195) -> (-145.205, -5.6203)
  line L578 (-148.507, 14.0004) -> (-148.507, 14.78019)
  line L579 (-130.405, 2.3007) -> (-129.632, 2.3007)
  line L580 (-131.206, -5.6203) -> (-131.206, -5.0195)
  line L581 (-146.006, -5.6203) -> (-146.006, -18.4195)
  line L582 (-131.206, -18.4195) -> (-130.405, -18.4195)
  line L583 (-131.206, -5.0195) -> (-145.205, -5.0195)
  line L584 (-131.207, 0.0297) -> (-131.207, 0.6305)
  line L585 (-146.782, 2.3007) -> (-146.007, 2.3007)
  line L586 (-148.507, 1.3) -> (-146.782, 1.3)
  line L587 (-151.806, 0.1795) -> (-148.507, 0.1795)
  line L588 (-148.507, 14.78019) -> (-151.806, 14.78019)
  line L589 (-122.107, 7.53034) -> (-122.982, 7.53034)
  line L590 (-122.982, 4.7302) -> (-122.107, 4.7302)
  line L591 (-137.022586, -19.279382) -> (-137.022586, -19.0203)
  line L592 (-16.6192, -56.5195) -> (-16.6192, -57.1203)
  line L593 (-2.61827, -43.7204) -> (-2.61827, -43.1196)
  line L594 (-146.782, 14.0004) -> (-148.507, 14.0004)
  arc A9 (0.156293, -56.6448) -> (-2.843707, -59.6448) centre (-2.843707, -56.6448) cw
  line L595 (-2.61827, -43.1196) -> (-16.6192, -43.1196)
  line L596 (0.156293, 13.555101) -> (0.156293, -56.6448)
  line L597 (-151.806, 14.0004) -> (-153.432, 14.0004)
  line L598 (-2.843707, -59.6448) -> (-240.231, -59.6448)
  arc A10 (-139.339414, -19.279382) -> (-137.022586, -19.279382) centre (-138.181, -21.4948) ccw
  line L599 (-145.205, -18.4195) -> (-145.205, -19.0203)
  line L600 (-240.231, 16.555101) -> (-2.843707, 16.555101)
  line L601 (-19.0004, -24.6704) -> (-19.7997, -24.6704)
  arc A11 (-240.231, -59.6448) -> (-243.231, -56.6448) centre (-240.231, -56.6448) cw
  line L602 (-145.205, -19.0203) -> (-139.339414, -19.0203)
  line L603 (-148.507, 0.1795) -> (-148.507, 1.3)
  line L604 (-16.6192, -43.1196) -> (-16.6192, -43.7204)
  line L605 (-130.405, -18.4195) -> (-130.405, -5.6203)
  line L606 (-16.6192, -57.1203) -> (-2.61827, -57.1203)
  line L607 (-104.725, 13.42971) -> (-105.525, 13.42971)
  line L608 (-17.4184, -43.7204) -> (-17.4184, -56.5195)
  line L609 (-153.432, 7.53034) -> (-154.307, 7.53034)
  line L610 (-154.307, 4.7302) -> (-153.432, 4.7302)
  line L611 (-129.632, 2.3007) -> (-129.632, 1.3)
  line L612 (-89.1494, 14.0004) -> (-89.1494, 12.99978)
  line L613 (-145.207, 0.0297) -> (-131.207, 0.0297)
  line L614 (-129.632, 14.0004) -> (-129.632, 12.99978)
  arc A12 (-2.843707, 16.555101) -> (0.156293, 13.555101) centre (-2.843707, 13.555101) cw
  line L615 (-145.207, 0.6305) -> (-145.207, 0.0297)
  line L616 (-153.432, 4.7302) -> (-153.432, 1.3)
  line L617 (-139.339414, -19.0203) -> (-139.339414, -19.279382)
  line L618 (-153.432, 14.0004) -> (-153.432, 7.53034)
  line L619 (-131.206, -19.0203) -> (-131.206, -18.4195)
  line L620 (-146.782, 1.3) -> (-146.782, 2.3007)
  line L621 (-146.006, -18.4195) -> (-145.205, -18.4195)
  line L622 (-2.61827, -57.1203) -> (-2.61827, -56.5195)
  line L623 (-16.6192, -43.7204) -> (-17.4184, -43.7204)
  line L624 (-40.7183, -57.1203) -> (-40.7183, -56.5195)
  line L625 (-20.828707, 13.42971) -> (-21.627707, 13.42971)
  line L626 (-45.4822, -24.6704) -> (-45.4822, -24.0696)
  line L627 (-59.4815, -24.6704) -> (-60.2823, -24.6704)
  line L628 (-45.4822, -24.0696) -> (-59.4815, -24.0696)
  line L629 (-59.4815, -24.0696) -> (-59.4815, -24.6704)
  line L630 (-69.0051, -18.4195) -> (-69.0051, -19.0203)
  line L631 (-59.4815, -38.0703) -> (-45.4822, -38.0703)
  line L632 (-69.8059, -18.4195) -> (-69.0051, -18.4195)
  line L633 (-35.9558, -5.0195) -> (-49.9551, -5.0195)
  line L634 (-59.4815, -37.4695) -> (-59.4815, -38.0703)
  line L635 (-69.0051, -19.0203) -> (-55.0058, -19.0203)
  line L636 (-69.0051, -5.6203) -> (-69.8059, -5.6203)
  line L637 (-40.4301, -38.0703) -> (-32.417127, -38.0703)
extrude "Extrude1" add sketch "minivan_universal_plate_mount" along normal blind 3 contours L2 A0 A9 L596 L598 L600 A11 A12 picked at (-212.59621, -52.784664) makes body 1
move_body "Move1" bodies 1 to x (1, 0, 0) y (0, 1, 0) z (0, 0, 1) at (40, 14, 0)
sketch "inner_walls" plane through (0, 0, 0) normal (0, 1, 0) x (1, 0, 0)
  line L0 (-124.231, 17.555101) -> (121.156293, 17.555101)
  line L1 (121.156293, 17.555101) -> (121.156293, -60.6448)
  line L2 (121.156293, -60.6448) -> (-124.231, -60.6448)
  line L3 (-124.231, -60.6448) -> (-124.231, 17.555101)
  line L4 (120.156293, -56.6448) -> (120.156293, 13.555101)
  line L5 (117.156293, 16.555101) -> (-120.231, 16.555101)
  line L6 (-120.231, -59.6448) -> (117.156293, -59.6448)
  line L7 (-123.231, 13.555101) -> (-123.231, -56.6448)
  dimension "d6" = 1
  dimension "d7" = 1
  dimension "d8" = 1
  dimension "d9" = 1
  constraint horizontal L0
  constraint vertical L1
  constraint horizontal L2
  constraint vertical L3
  measures "d6" distance of L1 L4
  measures "d7" distance of L0 L5
  measures "d8" distance of L2 L6
  measures "d9" distance of L3 L7
sketch "outer_walls" plane through (0, 0, 0) normal (0, 1, 0) x (1, 0, 0)
  line L0 (-129.231, 22.555101) -> (126.156293, 22.555101)
  line L1 (126.156293, 22.555101) -> (126.156293, -65.6448)
  line L2 (126.156293, -65.6448) -> (-129.231, -65.6448)
  line L3 (-129.231, -65.6448) -> (-129.231, 22.555101)
  line L4 (121.156293, 17.555101) -> (121.156293, -60.6448)
  line L5 (-124.231, 17.555101) -> (121.156293, 17.555101)
  line L6 (121.156293, -60.6448) -> (-124.231, -60.6448)
  line L7 (-124.231, -60.6448) -> (-124.231, 17.555101)
  dimension "d10" = 5
  dimension "d11" = 5
  dimension "d12" = 5
  dimension "d13" = 5
  constraint horizontal L0
  constraint vertical L1
  constraint horizontal L2
  constraint vertical L3
  measures "d10" distance of L1 L4
  measures "d11" distance of L0 L5
  measures "d12" distance of L2 L6
  measures "d13" distance of L3 L7
extrude "Extrude2" add sketch "outer_walls" along normal blind 22 separate body contours L0 L1 L2 L3 | L4 L5 L6 L7 picked at (39.360529, -63.978133) picked at (39.360529, -34.578166) makes body 2
shell "Shell1" thickness 4 removed faces 1 at (-44.101902, 22, 36.244833) on bodies 2
chamfer "Chamfer1" distance 5 angle 45 4 edges at (-1.537353, 0, 65.6448) (-129.231, 0, 21.54485) (-1.537353, 0, -22.555101) (126.156293, 0, 21.544849) on bodies 2